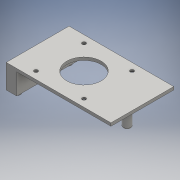
# Autodesk Inventor part: MotorKuggHolder
Saved by Autodesk Inventor 2016 (Build 200138000, 138)
## iProperties
Created: 2018-03-03
Part Number: MotorKuggHolder
Material: Generic
Document SubType Name: Modeling
Designer: Simon
Density: 1 g/cm^3
Appearance: Default
Author: Simon
Autodesk Inventor part; units mm, degrees
ref_plane "YZ Plane" through (0, 0, 0) normal (1, 0, 0) x (0, 1, 0)
sketch "Sketch1" plane through (0, 0, 0) normal (0, 0, 1) x (1, 0, 0)
  line L0 (0, 0) -> (60, 0)
  line L1 (60, 0) -> (60, 42)
  line L2 (60, 42) -> (0, 42)
  line L3 (0, 42) -> (0, 0)
  line L4 (0, 42) -> (0, 0)
  dimension "d0" = 60
  dimension "d1" = 42
  constraints: 10 end point, 2 parallel, 1 horizontal, 1 perpendicular
  measures "d0" distance of L2.end L1.end
  measures "d1" distance of L1.end L0.end
extrude "Extrusion1" add sketch "Sketch1" along normal blind 2
sketch "Sketch2" plane through (0, 0, 2) normal (0, 0, 1) x (1, 0, 0)
  circle A0 centre (21, 21) radius 11.5
  line L0 (0, 42) -> (0, 0) projected
  line L1 (60, 42) -> (0, 42) projected
  dimension "d6" = 23
  dimension "d7" = 21
  dimension "d8" = 21
  constraints: 1 centre point
  measures "d6" diameter of A0
  measures "d7" distance from line of L0 A0.centre
  measures "d8" distance from line of L1 A0.centre
extrude "Extrusion2" cut sketch "Sketch2" against normal blind 2
sketch "Sketch3" plane through (0, 0, 0) normal (0, 0, -1) x (-1, 0, 0)
  circle A0 centre (-4.95, 4.95) radius 1.25
  line L0 (0, 0) -> (-60, 0) projected
  line L1 (0, 42) -> (0, 0) projected
  dimension "d12" = 3.7
  dimension "d13" = 2.5
  dimension "d14" = 3.7
  constraints: 1 centre point
  measures "d12" distance edge to line of A0 L0
  measures "d13" diameter of A0
  measures "d14" distance edge to line of A0 L1
ref_plane "Work Plane2" through (0, 21, 0) normal (0, -1, 0) x (1, 0, 0)
extrude "Extrusion3" cut sketch "Sketch3" against normal through all
mirror "Mirror1" about plane through (0, 21, 0) normal (0, -1, 0) of "Extrusion3"
ref_plane "Work Plane4" through (21, 0, 0) normal (-1, 0, 0) x (0, 0, 1)
mirror "Mirror2" about plane through (21, 0, 0) normal (-1, 0, 0) of "Extrusion3", "Mirror1"
sketch "Sketch4" plane through (0, 0, 0) normal (0, 0, -1) x (-1, 0, 0)
  circle A0 centre (-21, 21) radius 11.5 projected
  circle A1 centre (-49.8, 21) radius 2.5
  point P0 (0, 0)
  dimension "d20" = 5
  dimension "d21" = 28.8
  constraints: 1 centre point
  measures "d20" diameter of A1
  measures "d21" distance of A1.centre A0.centre
extrude "Extrusion4" add sketch "Sketch4" along normal blind 16 contours A1
fillet "Fillet2" radius 1 1 edges at (52.3, 21, -16)
sketch "Sketch5" plane through (0, 0, 0) normal (-1, 0, 0) x (0, 0, 1)
  line L0 (0, 42) -> (0, 0) projected
  line L1 (0, 42) -> (2, 42) projected
  line L2 (0, 0) -> (2, 0)
  line L3 (2, 0) -> (2, 42)
  line L4 (2, 42) -> (0, 42)
  line L5 (0, 42) -> (0, 0)
  constraints: 8 end point, 2 parallel, 1 horizontal, 1 perpendicular
extrude "Extrusion5" add sketch "Sketch5" along normal blind 10
sketch "Sketch6" plane through (0, 0, 0) normal (0, 0, -1) x (-1, 0, 0)
  line L0 (10, 42) -> (10, 0) projected
  line L1 (-60, 42) -> (10, 42) projected
  line L2 (10, 0) -> (3, 0)
  line L3 (3, 0) -> (3, 42)
  line L4 (3, 42) -> (10, 42)
  line L5 (10, 42) -> (10, 0)
  point P0 (0, 0)
  dimension "d32" = 7
  constraints: 8 end point, 2 parallel, 1 horizontal, 1 perpendicular, 1 point on line
  measures "d32" distance of L3.end L4.end
extrude "Extrusion6" add sketch "Sketch6" along normal blind 14
sketch "Sketch7" plane through (0, 0, -14) normal (0, 0, -1) x (-1, 0, 0)
  circle A0 centre (6.5, 4) radius 2
  line L0 (3, 42) -> (3, 0) projected
  line L1 (3, 0) -> (10, 0) projected
  circle A1 centre (6.5, 21) radius 2
  circle A2 centre (6.5, 38) radius 2
  point P0 (0, 0)
  dimension "d35" = 4
  dimension "d36" = 3.5
  dimension "d37" = 4
  dimension "d40" = 17
  constraints: 3 centre point, 1 vertical, 4 other
  measures "d35" diameter of A0
  measures "d36" distance from line of L0 A0.centre
  measures "d37" distance from line of L1 A0.centre
  measures "d40" distance of A0.centre A1.centre
extrude "Extrusion7" add sketch "Sketch7" along normal blind 2
chamfer "Chamfer2" distance 1 angle 45 2 edges at (35.8, 4.95, 0) (35.8, 37.05, 0)
sketch "Sketch9" plane through (0, 0, 0) normal (0, 0, -1) x (-1, 0, 0)
  circle A0 centre (-4.95, 4.95) radius 1.25 projected
  circle A1 centre (-4.95, 37.05) radius 1.25 projected
  circle A2 centre (-4.95, 4.95) radius 2.5
  circle A3 centre (-4.95, 37.05) radius 2.5
  point P0 (0, 0)
  dimension "d50" = 5
  dimension "d51" = 5
  constraints: 2 centre point, 2 coincident
  measures "d50" diameter of A2
  measures "d51" diameter of A3
extrude "Extrusion8" add sketch "Sketch9" along normal blind 2
fillet "Fillet3" radius 2 2 edges at (7.45, 4.95, 0) (7.45, 37.05, 0)
body "Solid1"
